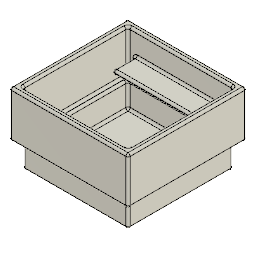
Component Storage v3 (Autodesk Fusion 360 design; units mm, degrees)
Autodesk Fusion 360 part; units mm, degrees
sketch "Sketch1" plane through (0, 0, 0) normal (0, 0, 1) x (1, 0, 0)
  line L0 (13.0969, -13.0969) -> (-13.0969, -13.0969)
  line L1 (-13.0969, -13.0969) -> (-13.0969, 13.0969)
  line L2 (-13.0969, 13.0969) -> (13.0969, 13.0969)
  line L3 (13.0969, 13.0969) -> (13.0969, -13.0969)
  line L4 (13.0969, -13.0969) -> (-13.0969, 13.0969) construction
  line L5 (-13.0969, -13.0969) -> (13.0969, 13.0969) construction
  line L6 (11.5969, -11.5969) -> (-11.5969, -11.5969)
  line L7 (-11.5969, -11.5969) -> (-11.5969, 11.5969)
  line L8 (-11.5969, 11.5969) -> (11.5969, 11.5969)
  line L9 (11.5969, 11.5969) -> (11.5969, -11.5969)
  line L10 (-10.5969, -10.5969) -> (-10.5969, 10.5969)
  line L11 (-10.5969, 10.5969) -> (10.5969, 10.5969)
  line L12 (10.5969, 10.5969) -> (10.5969, -10.5969)
  line L13 (10.5969, -10.5969) -> (-10.5969, -10.5969)
  dimension "d7" = 26.1938
  dimension "d8" = 26.1938
  dimension "d10" = 1.5
  dimension "d18" = 2.5
  constraint horizontal L0
  constraint perpendicular L0 L1
  constraint parallel L0 L2
  constraint parallel L1 L3
  constraint coincident L4 origin
  constraint coincident L5 origin
  measures "d7" distance of L1.end L2.end
  measures "d8" distance of L0.end L1.end
extrude "Extrude1" add sketch "Sketch1" along normal blind 15.8083 contours L0 L1 L2 L3
extrude "Extrude2" add sketch "Sketch1" along normal blind 1 contours L6 L7 L8 L9 | L10 L11 L12 L13
extrude "Extrude3" [suppressed]
extrude "Extrude4" add sketch "Sketch1" along normal blind 6.5 contours L6 L7 L8 L9
extrude "Extrude5" cut sketch "Sketch1" along normal blind 5.5 contours L0 L1 L2 L3
sketch "Sketch2" plane through (0, 11.5969, 0) normal (0, -1, 0) x (1, 0, 0)
  line L0 (-11.5969, 6.5) -> (11.5969, 6.5)
  line L1 (11.5969, 6.5) -> (11.5969, 15.8083)
  line L2 (11.5969, 15.8083) -> (-11.5969, 15.8083)
  line L3 (-11.5969, 15.8083) -> (-11.5969, 6.5)
  line L4 (-10, 10.8083) -> (10, 10.8083)
  line L5 (10, 10.8083) -> (10, 9.8083)
  line L6 (10, 9.8083) -> (-10, 9.8083)
  line L7 (-10, 9.8083) -> (-10, 10.8083)
  line L8 (0, 15.8083) -> (0, 10.8083) construction
  point P0 (0, 10.8083)
  point P1 (0, 10.8083)
  dimension "d26" = 20
  dimension "d27" = 1
  dimension "d30" = 5
  constraint horizontal L4
  constraint vertical L5
  constraint horizontal L6
  constraint vertical L7
  constraint midpoint L4 P1
  constraint coincident P1 P0
  constraint midpoint L2 L8.start
  constraint perpendicular L2 L8
  measures "d26" distance of L4.start L4.end
  measures "d27" distance of L4.start L6.end
  measures "d30" distance of L8.start P1
extrude "Extrude6" add sketch "Sketch2" along normal blind 5 contours L4 L5 L6 L7
fillet "Fillet1" radius 0.4762 26 faces at (4.3656, -13.0969, 12.3722) (-11.5969, -3.8656, 12.7056) (-4.3656, 13.0969, 8.9361) (-3.8656, 3.8656, 0) (3.8656, -11.5969, 1.8333) (-13.0969, -4.3656, 8.9361) (3.5323, -10.5969, 2.8333) (-3.5323, 3.5323, 1) (-10.5969, -3.5323, 2.8333) (11.2635, -3.5323, 6.5) (12.5969, -3.8656, 15.8083) (-3.3333, 6.5969, 10.475) (-3.3333, 9.9302, 10.8083) (12.5969, -3.8656, 5.5) (-3.5323, 10.5969, 2.8333) (3.3333, 11.5969, 14.1417) (10.5969, 3.5323, 2.8333) (3.3333, 8.2635, 9.8083) (13.0969, 4.3656, 8.9361) (11.5969, 3.8656, 3.6667) (-3.8656, -11.5969, 12.7056) (-3.8656, 11.5969, 3.6667) (11.5969, -3.8656, 9.6028) (-10, 9.9302, 10.1417) (-11.5969, -3.8656, 1.8333) (10, 9.9302, 10.475)
equation "boxiw = 8.25 in" comment "Internal width of larger container"
equation "boxil = 8.25 in" comment "Internal length of larger container"
equation "cupnumw = 8" comment "Number of cups along the width of the box"
equation "cupw = boxiw / cupnumw"
equation "cupl = boxil / cupnuml"
equation "cupnuml = 8" comment "Number of cups along the length of the box"
equation "d7 = cupw"
equation "d8 = cupl"
equation "thick = 1 mm" comment "Thickness of the cups' parts"
equation "d10 = thick + tol"
equation "boxih = 2.75 in" comment "Internal height of larger container"
equation "cupnumh = 6" comment "Number of cups along the height of the box"
equation "cuph = ( boxih + overlap * ( cupnumh - 1 ) ) / cupnumh"
equation "d14 = cuph"
equation "d16 = thick"
equation "d18 = thick * 2 + tol"
equation "d19 = mm"
equation "overlap = 5 mm"
equation "d22 = overlap + thick + tol"
equation "d24 = overlap + tol"
equation "d27 = thick"
equation "d30 = overlap"
equation "d32 = thick / 2.1"
equation "tol = 0.5 mm"
